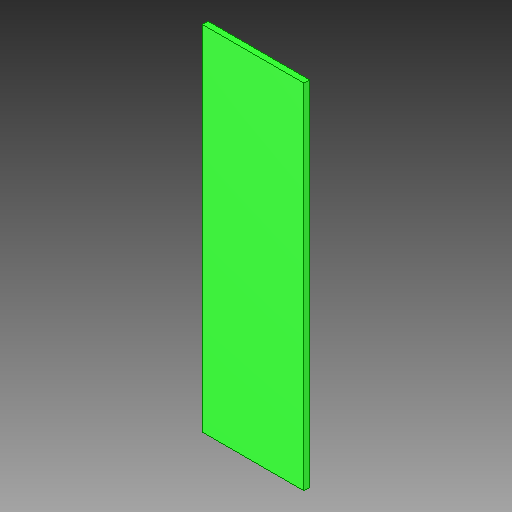
# Autodesk Inventor part: TEENSY_3_5_ALL_PINS
Saved by Autodesk Inventor 2017 (Build 210142000, 142)
## iProperties
Created: 2019-06-13
Part Number: TEENSY_3_5_ALL_PINS
Material: Generic
Document SubType Name: Modeling
Designer: Marc
Density: 1 g/cm^3
Appearance: TEENSY_3_5_ALL_PINS, TEENSY_3_5_ALL_PINS
Author: Marc
Autodesk Inventor part; units mm, degrees
ref_plane "YZ Plane" through (0, 0, 0) normal (1, 0, 0) x (0, 1, 0)
ref_plane "XZ Plane" through (0, 0, 0) normal (0, 1, 0) x (-1, 0, 0)
ref_plane "XY Plane" through (0, 0, 0) normal (0, 0, 1) x (1, 0, 0)
sketch "TEENSY_3_5_ALL_PINS, TEENSY_3_5_ALL_PINS_63" plane through (0, 0, 0) normal (0, 0, 1) x (1, 0, 0)
  line L0 (-8.9535, 33.02) -> (8.9535, 33.02)
  line L1 (8.9535, 33.02) -> (8.9535, -29.21)
  line L2 (8.9535, -29.21) -> (-8.9535, -29.21)
  line L3 (-8.9535, -29.21) -> (-8.9535, 33.02)
  constraints: 8 end point
extrude "Extrusion1" add sketch "TEENSY_3_5_ALL_PINS, TEENSY_3_5_ALL_PINS_63" along normal blind 1
body "Solid1"
